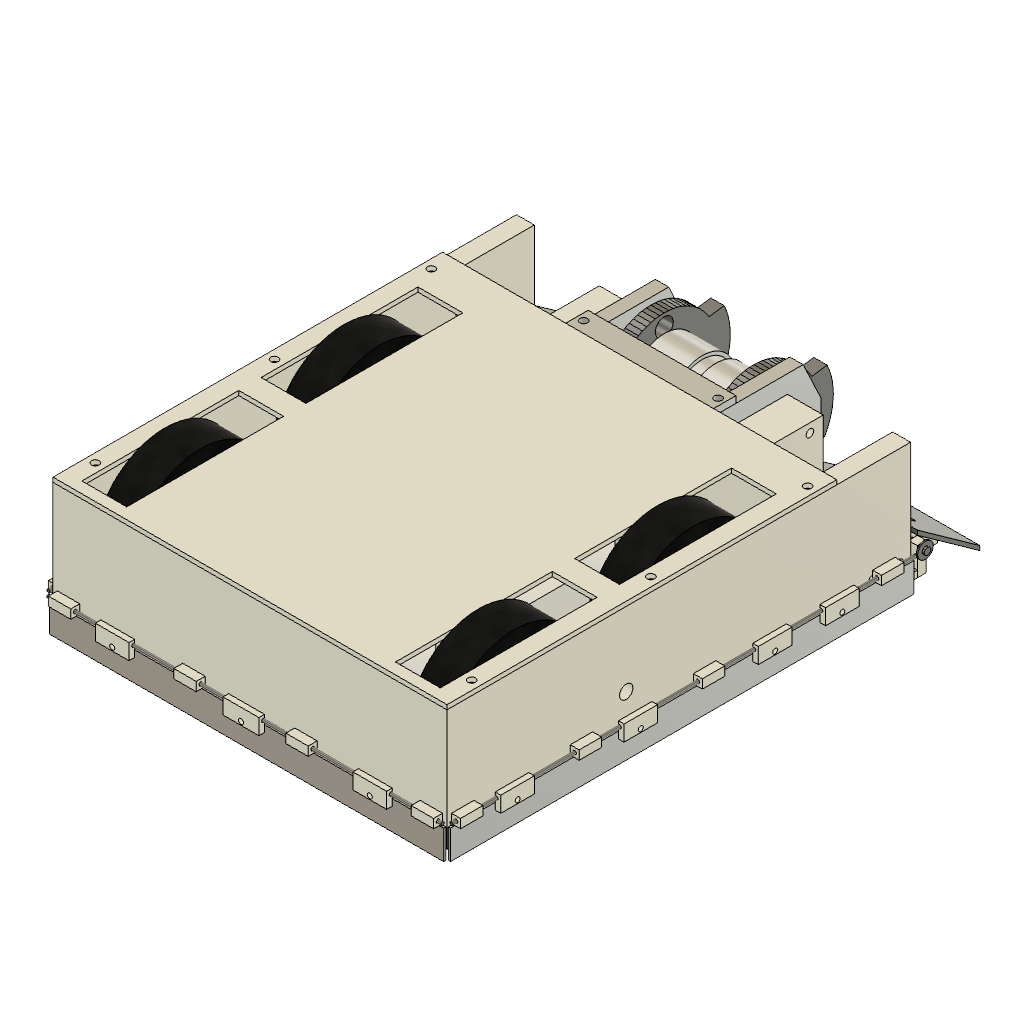
ROBOT_V4_Beater (Autodesk Fusion 360 design; units mm, degrees)
part number: 2026-10-03-23-02-07-533
part number: 2026-10-03-23-02-07-742
part number: 2026-10-03-23-02-07-825
part number: 2026-10-03-23-02-08-845
part number: 2026-10-03-23-02-09-094
part number: 2026-10-03-23-02-09-103
part number: 2026-10-03-23-02-09-172
part number: 2026-10-03-23-02-09-236
part number: 2026-10-03-23-02-09-311
part number: 2026-10-03-23-02-09-393
part number: 2026-10-03-23-02-09-746
part number: 2026-10-03-23-02-10-052
part number: 2026-10-03-23-02-10-324
part number: 2026-10-03-23-02-10-365
part number: 2026-10-03-23-02-10-407
part number: 2026-10-03-23-02-10-450
part number: 2026-10-03-23-02-10-494
part number: 2026-10-03-23-02-10-539
part number: 2026-10-03-23-02-10-582
part number: 2026-10-03-23-02-10-687
part number: 2026-10-03-23-02-10-740
part number: 2026-10-03-23-02-10-976
part number: 2026-10-03-23-02-11-027
part number: 2026-10-03-23-02-11-079
part number: 2026-10-03-23-02-11-094
part number: 2026-10-03-23-02-11-260
part number: 2026-10-03-23-02-11-385
part number: 2026-10-03-23-02-11-847
part number: 2026-10-03-23-02-12-017
part number: 2026-10-03-23-02-12-191
part number: 2026-10-03-23-02-12-302
part number: 2026-10-03-23-02-12-373
part number: 2026-10-03-23-02-12-902
part number: 2026-10-03-23-02-13-104
part number: 2026-10-03-23-02-14-285
part number: 2026-10-03-23-02-14-424
part number: 2026-10-03-23-02-14-508
part number: 2026-10-03-23-02-14-531
part number: 2026-10-03-23-02-14-614
part number: 2026-10-03-23-02-15-140
part number: 2026-10-03-23-02-15-408
part number: 2026-10-03-23-02-15-682
part number: 2026-10-03-23-02-15-969
part number: 2026-10-03-23-02-16-272
part number: 2026-10-03-23-02-16-375
part number: 2026-10-03-23-02-16-912
part number: 2026-10-03-23-02-17-232
part number: 2026-10-03-23-02-17-564
part number: 2026-10-03-23-02-17-904
part number: 2026-10-03-23-02-18-255
part number: 2026-10-03-23-02-18-371
part number: 2026-10-03-23-02-19-002
part number: 2026-10-03-23-02-19-385
part number: 2026-10-03-23-02-19-768
part number: 2026-10-03-23-02-20-163
part number: 2026-10-03-23-02-20-204
part number: 2026-10-03-23-02-20-339
part number: 2026-10-03-23-02-20-844
part number: 2026-10-03-23-02-20-994
part number: 2026-10-03-23-02-21-141
part number: 2026-10-03-23-02-21-679
part number: 2026-10-03-23-02-21-843
part number: 2026-10-03-23-02-22-015
part number: 2026-10-03-23-02-22-630
part number: 2026-10-03-23-02-22-845
part number: 2026-10-03-23-02-23-035
part number: 2026-10-03-23-02-23-656
part number: 2026-10-03-23-02-23-827
part number: 2026-10-03-23-02-23-873
part number: 2026-10-03-23-02-24-050
part number: 2026-10-03-23-02-24-210
part number: 2026-10-03-23-02-24-370
part number: 2026-10-03-23-02-24-531
part number: 2026-10-03-23-02-24-696
part number: 2026-10-03-23-02-24-861
part number: 2026-10-03-23-02-25-025
part number: 2026-10-03-23-02-25-193
part number: 2026-10-03-23-02-25-361
Autodesk Fusion 360 part; units mm, degrees
(part 1 of 3)
sketch "Sketch1" plane through (0, 0, 0) normal (0, 1, 0) x (1, 0, 0) in component "Tub_TPU"
  line L0 (-88, -110) -> (88, -110)
  line L1 (88, -110) -> (88, 64)
  line L2 (88, 64) -> (-88, 64)
  line L3 (-88, 64) -> (-88, -110)
extrude "Extrude1" add sketch "Sketch1" along normal blind 3 from surface at 4 makes body 1 in component "Tub_TPU"
sketch "Floor_WheelWell" plane through (0, 0, 0) normal (1, 0, 0) x (0, 0, -1) in component "Tub_TPU"
  line L0 (-25, 3) -> (-25, 8)
  line L1 (-25, 8) -> (45, 8)
  line L2 (45, 8) -> (45, 3)
  line L3 (45, 3) -> (-25, 3)
extrude "Extrude2" cut sketch "Floor_WheelWell" along normal blind 20 from surface at -80 bodies 1 in component "Tub_TPU"
sketch "Floor_WheelWell (1)" plane through (0, 0, 0) normal (1, 0, 0) x (0, 0, -1) in component "Tub_TPU"
  line L0 (-105, 3) -> (-105, 8)
  line L1 (-105, 8) -> (-35, 8)
  line L2 (-35, 8) -> (-35, 3)
  line L3 (-35, 3) -> (-105, 3)
extrude "Extrude3" cut sketch "Floor_WheelWell (1)" along normal blind 20 from surface at -80 bodies 1 in component "Tub_TPU"
sketch "Floor_WheelWell (2)" plane through (0, 0, 0) normal (1, 0, 0) x (0, 0, -1) in component "Tub_TPU"
  line L0 (-25, 3) -> (-25, 8)
  line L1 (-25, 8) -> (45, 8)
  line L2 (45, 8) -> (45, 3)
  line L3 (45, 3) -> (-25, 3)
extrude "Extrude4" cut sketch "Floor_WheelWell (2)" along normal blind 20 from surface at 60 bodies 1 in component "Tub_TPU"
sketch "Floor_WheelWell (3)" plane through (0, 0, 0) normal (1, 0, 0) x (0, 0, -1) in component "Tub_TPU"
  line L0 (-105, 3) -> (-105, 8)
  line L1 (-105, 8) -> (-35, 8)
  line L2 (-35, 8) -> (-35, 3)
  line L3 (-35, 3) -> (-105, 3)
extrude "Extrude5" cut sketch "Floor_WheelWell (3)" along normal blind 20 from surface at 60 bodies 1 in component "Tub_TPU"
sketch "Side_Wall" plane through (0, 0, 0) normal (1, 0, 0) x (0, 0, -1) in component "Tub_TPU"
  line L0 (-110, 7) -> (-110, 58)
  line L1 (-110, 58) -> (97, 58)
  line L2 (97, 58) -> (97, 7)
  line L3 (97, 7) -> (-110, 7)
extrude "Extrude6" add sketch "Side_Wall" along normal blind 8 from surface at -88 bodies 1 in component "Tub_TPU"
sketch "Side_Wall (1)" plane through (0, 0, 0) normal (1, 0, 0) x (0, 0, -1) in component "Tub_TPU"
  line L0 (-110, 7) -> (-110, 58)
  line L1 (-110, 58) -> (97, 58)
  line L2 (97, 58) -> (97, 7)
  line L3 (97, 7) -> (-110, 7)
extrude "Extrude7" add sketch "Side_Wall (1)" along normal blind 8 from surface at 80 bodies 1 in component "Tub_TPU"
sketch "Rear_Wall" plane through (0, 0, 0) normal (1, 0, 0) x (0, 0, -1) in component "Tub_TPU"
  line L0 (-110, 7) -> (-110, 58)
  line L1 (-110, 58) -> (-104, 58)
  line L2 (-104, 58) -> (-104, 7)
  line L3 (-104, 7) -> (-110, 7)
extrude "Extrude8" add sketch "Rear_Wall" along normal blind 160 from surface at -80 bodies 1 in component "Tub_TPU"
sketch "Front_Bulkhead" plane through (0, 0, 0) normal (1, 0, 0) x (0, 0, -1) in component "Tub_TPU"
  line L0 (62, 7) -> (62, 58)
  line L1 (62, 58) -> (64, 58)
  line L2 (64, 58) -> (64, 7)
  line L3 (64, 7) -> (62, 7)
extrude "Extrude9" add sketch "Front_Bulkhead" along normal blind 160 from surface at -80 bodies 1 in component "Tub_TPU"
sketch "Belt_Slot" plane through (0, 0, 0) normal (1, 0, 0) x (0, 0, -1) in component "Tub_TPU"
  line L0 (61, 12) -> (61, 52)
  line L1 (61, 52) -> (65, 52)
  line L2 (65, 52) -> (65, 12)
  line L3 (65, 12) -> (61, 12)
extrude "Extrude10" cut sketch "Belt_Slot" along normal blind 12 from surface at -6 bodies 1 in component "Tub_TPU"
sketch "Motor_Wall" plane through (0, 0, 0) normal (1, 0, 0) x (0, 0, -1) in component "Tub_TPU"
  line L0 (-3, 7) -> (-3, 58)
  line L1 (-3, 58) -> (23, 58)
  line L2 (23, 58) -> (23, 7)
  line L3 (23, 7) -> (-3, 7)
extrude "Extrude11" add sketch "Motor_Wall" along normal blind 4 from surface at -60 bodies 1 in component "Tub_TPU"
sketch "Motor_Wall (1)" plane through (0, 0, 0) normal (1, 0, 0) x (0, 0, -1) in component "Tub_TPU"
  line L0 (-3, 7) -> (-3, 58)
  line L1 (-3, 58) -> (23, 58)
  line L2 (23, 58) -> (23, 7)
  line L3 (23, 7) -> (-3, 7)
extrude "Extrude12" add sketch "Motor_Wall (1)" along normal blind 4 from surface at 56 bodies 1 in component "Tub_TPU"
sketch "Motor_Shaft_Hole" plane through (0, 0, 0) normal (1, 0, 0) x (0, 0, -1) in component "Tub_TPU"
  circle A0 centre (10, 32) radius 4
extrude "Extrude13" cut sketch "Motor_Shaft_Hole" along normal blind 6 from surface at -61 bodies 1 in component "Tub_TPU"
sketch "Motor_Shaft_Hole (1)" plane through (0, 0, 0) normal (1, 0, 0) x (0, 0, -1) in component "Tub_TPU"
  circle A0 centre (10, 32) radius 4
extrude "Extrude14" cut sketch "Motor_Shaft_Hole (1)" along normal blind 6 from surface at 55 bodies 1 in component "Tub_TPU"
sketch "Motor_Wall (2)" plane through (0, 0, 0) normal (1, 0, 0) x (0, 0, -1) in component "Tub_TPU"
  line L0 (-83, 7) -> (-83, 58)
  line L1 (-83, 58) -> (-57, 58)
  line L2 (-57, 58) -> (-57, 7)
  line L3 (-57, 7) -> (-83, 7)
extrude "Extrude15" add sketch "Motor_Wall (2)" along normal blind 4 from surface at -60 bodies 1 in component "Tub_TPU"
sketch "Motor_Wall (3)" plane through (0, 0, 0) normal (1, 0, 0) x (0, 0, -1) in component "Tub_TPU"
  line L0 (-83, 7) -> (-83, 58)
  line L1 (-83, 58) -> (-57, 58)
  line L2 (-57, 58) -> (-57, 7)
  line L3 (-57, 7) -> (-83, 7)
extrude "Extrude16" add sketch "Motor_Wall (3)" along normal blind 4 from surface at 56 bodies 1 in component "Tub_TPU"
sketch "Motor_Shaft_Hole (2)" plane through (0, 0, 0) normal (1, 0, 0) x (0, 0, -1) in component "Tub_TPU"
  circle A0 centre (-70, 32) radius 4
extrude "Extrude17" cut sketch "Motor_Shaft_Hole (2)" along normal blind 6 from surface at -61 bodies 1 in component "Tub_TPU"
sketch "Motor_Shaft_Hole (3)" plane through (0, 0, 0) normal (1, 0, 0) x (0, 0, -1) in component "Tub_TPU"
  circle A0 centre (-70, 32) radius 4
extrude "Extrude18" cut sketch "Motor_Shaft_Hole (3)" along normal blind 6 from surface at 55 bodies 1 in component "Tub_TPU"
sketch "Front_Floor" plane through (0, 0, 0) normal (1, 0, 0) x (0, 0, -1) in component "Tub_TPU"
  line L0 (64, 4) -> (64, 7)
  line L1 (64, 7) -> (100, 7)
  line L2 (100, 7) -> (100, 4)
  line L3 (100, 4) -> (64, 4)
extrude "Extrude19" add sketch "Front_Floor" along normal blind 54 from surface at -88 bodies 1 in component "Tub_TPU"
sketch "Front_Floor (1)" plane through (0, 0, 0) normal (1, 0, 0) x (0, 0, -1) in component "Tub_TPU"
  line L0 (64, 4) -> (64, 7)
  line L1 (64, 7) -> (100, 7)
  line L2 (100, 7) -> (100, 4)
  line L3 (100, 4) -> (64, 4)
extrude "Extrude20" add sketch "Front_Floor (1)" along normal blind 54 from surface at 34 bodies 1 in component "Tub_TPU"
sketch "Block_Screw_Clearance" plane through (0, 0, 0) normal (1, 0, 0) x (0, 0, -1) in component "Tub_TPU"
  circle A0 centre (80, 13.5) radius 1.7
extrude "Extrude21" cut sketch "Block_Screw_Clearance" along normal blind 10 from surface at -89 bodies 1 in component "Tub_TPU"
sketch "Block_Screw_Clearance (1)" plane through (0, 0, 0) normal (1, 0, 0) x (0, 0, -1) in component "Tub_TPU"
  circle A0 centre (92, 13.5) radius 1.7
extrude "Extrude22" cut sketch "Block_Screw_Clearance (1)" along normal blind 10 from surface at -89 bodies 1 in component "Tub_TPU"
sketch "Block_Screw_Clearance (2)" plane through (0, 0, 0) normal (1, 0, 0) x (0, 0, -1) in component "Tub_TPU"
  circle A0 centre (80, 13.5) radius 1.7
extrude "Extrude23" cut sketch "Block_Screw_Clearance (2)" along normal blind 10 from surface at 79 bodies 1 in component "Tub_TPU"
sketch "Block_Screw_Clearance (3)" plane through (0, 0, 0) normal (1, 0, 0) x (0, 0, -1) in component "Tub_TPU"
  circle A0 centre (92, 13.5) radius 1.7
extrude "Extrude24" cut sketch "Block_Screw_Clearance (3)" along normal blind 10 from surface at 79 bodies 1 in component "Tub_TPU"
sketch "Weapon_Side_Block" plane through (0, 0, 0) normal (1, 0, 0) x (0, 0, -1) in component "Tub_TPU"
  line L0 (64, 7) -> (64, 50)
  line L1 (64, 50) -> (96, 50)
  line L2 (96, 50) -> (96, 7)
  line L3 (96, 7) -> (64, 7)
extrude "Extrude25" add sketch "Weapon_Side_Block" along normal blind 16 from surface at -50 bodies 1 in component "Tub_TPU"
sketch "Upright_Screw_Clearance" plane through (0, 0, 0) normal (1, 0, 0) x (0, 0, -1) in component "Tub_TPU"
  circle A0 centre (70, 14) radius 1.7
extrude "Extrude26" cut sketch "Upright_Screw_Clearance" along normal blind 18 from surface at -51 bodies 1 in component "Tub_TPU"
sketch "Upright_Screw_Clearance (1)" plane through (0, 0, 0) normal (1, 0, 0) x (0, 0, -1) in component "Tub_TPU"
  circle A0 centre (70, 50) radius 1.7
extrude "Extrude27" cut sketch "Upright_Screw_Clearance (1)" along normal blind 18 from surface at -51 bodies 1 in component "Tub_TPU"
sketch "Upright_Screw_Clearance (2)" plane through (0, 0, 0) normal (1, 0, 0) x (0, 0, -1) in component "Tub_TPU"
  circle A0 centre (90, 14) radius 1.7
extrude "Extrude28" cut sketch "Upright_Screw_Clearance (2)" along normal blind 18 from surface at -51 bodies 1 in component "Tub_TPU"
sketch "Upright_Screw_Clearance (3)" plane through (0, 0, 0) normal (1, 0, 0) x (0, 0, -1) in component "Tub_TPU"
  circle A0 centre (90, 46) radius 1.7
extrude "Extrude29" cut sketch "Upright_Screw_Clearance (3)" along normal blind 18 from surface at -51 bodies 1 in component "Tub_TPU"
sketch "Weapon_Side_Block (1)" plane through (0, 0, 0) normal (1, 0, 0) x (0, 0, -1) in component "Tub_TPU"
  line L0 (64, 7) -> (64, 50)
  line L1 (64, 50) -> (96, 50)
  line L2 (96, 50) -> (96, 7)
  line L3 (96, 7) -> (64, 7)
extrude "Extrude30" add sketch "Weapon_Side_Block (1)" along normal blind 16 from surface at 34 bodies 1 in component "Tub_TPU"
sketch "Upright_Screw_Clearance (4)" plane through (0, 0, 0) normal (1, 0, 0) x (0, 0, -1) in component "Tub_TPU"
  circle A0 centre (70, 14) radius 1.7
extrude "Extrude31" cut sketch "Upright_Screw_Clearance (4)" along normal blind 18 from surface at 33 bodies 1 in component "Tub_TPU"
sketch "Upright_Screw_Clearance (5)" plane through (0, 0, 0) normal (1, 0, 0) x (0, 0, -1) in component "Tub_TPU"
  circle A0 centre (70, 50) radius 1.7
extrude "Extrude32" cut sketch "Upright_Screw_Clearance (5)" along normal blind 18 from surface at 33 bodies 1 in component "Tub_TPU"
sketch "Upright_Screw_Clearance (6)" plane through (0, 0, 0) normal (1, 0, 0) x (0, 0, -1) in component "Tub_TPU"
  circle A0 centre (90, 14) radius 1.7
extrude "Extrude33" cut sketch "Upright_Screw_Clearance (6)" along normal blind 18 from surface at 33 bodies 1 in component "Tub_TPU"
sketch "Upright_Screw_Clearance (7)" plane through (0, 0, 0) normal (1, 0, 0) x (0, 0, -1) in component "Tub_TPU"
  circle A0 centre (90, 46) radius 1.7
extrude "Extrude34" cut sketch "Upright_Screw_Clearance (7)" along normal blind 18 from surface at 33 bodies 1 in component "Tub_TPU"
sketch "Lid_Insert" plane through (0, 0, 0) normal (0, 1, 0) x (1, 0, 0) in component "Tub_TPU"
  circle A0 centre (-84, -95) radius 2
extrude "Extrude35" cut sketch "Lid_Insert" along normal blind 8 from surface at 51 bodies 1 in component "Tub_TPU"
sketch "Lid_Insert (1)" plane through (0, 0, 0) normal (0, 1, 0) x (1, 0, 0) in component "Tub_TPU"
  circle A0 centre (-84, -15) radius 2
extrude "Extrude36" cut sketch "Lid_Insert (1)" along normal blind 8 from surface at 51 bodies 1 in component "Tub_TPU"
sketch "Lid_Insert (2)" plane through (0, 0, 0) normal (0, 1, 0) x (1, 0, 0) in component "Tub_TPU"
  circle A0 centre (-84, 55) radius 2
extrude "Extrude37" cut sketch "Lid_Insert (2)" along normal blind 8 from surface at 51 bodies 1 in component "Tub_TPU"
sketch "Lid_Insert (3)" plane through (0, 0, 0) normal (0, 1, 0) x (1, 0, 0) in component "Tub_TPU"
  circle A0 centre (84, -95) radius 2
extrude "Extrude38" cut sketch "Lid_Insert (3)" along normal blind 8 from surface at 51 bodies 1 in component "Tub_TPU"
sketch "Lid_Insert (4)" plane through (0, 0, 0) normal (0, 1, 0) x (1, 0, 0) in component "Tub_TPU"
  circle A0 centre (84, -15) radius 2
extrude "Extrude39" cut sketch "Lid_Insert (4)" along normal blind 8 from surface at 51 bodies 1 in component "Tub_TPU"
sketch "Lid_Insert (5)" plane through (0, 0, 0) normal (0, 1, 0) x (1, 0, 0) in component "Tub_TPU"
  circle A0 centre (84, 55) radius 2
extrude "Extrude40" cut sketch "Lid_Insert (5)" along normal blind 8 from surface at 51 bodies 1 in component "Tub_TPU"
sketch "Switch_Key_Hole" plane through (0, 0, 0) normal (1, 0, 0) x (0, 0, -1) in component "Tub_TPU"
  circle A0 centre (-30, 25) radius 3
extrude "Extrude41" cut sketch "Switch_Key_Hole" along normal blind 10 from surface at 79 bodies 1 in component "Tub_TPU"
sketch "Sketch1 (2)" plane through (0, 0, 0) normal (0, 1, 0) x (1, 0, 0) in component "Lid_TPU_2mm"
  line L0 (-88, -110) -> (88, -110)
  line L1 (88, -110) -> (88, 64)
  line L2 (88, 64) -> (-88, 64)
  line L3 (-88, 64) -> (-88, -110)
extrude "Extrude1'" add sketch "Sketch1 (2)" along normal blind 2 from surface at 58 separate body makes body 2 in component "Lid_TPU_2mm"
sketch "Lid_WheelWell" plane through (0, 0, 0) normal (1, 0, 0) x (0, 0, -1) in component "Lid_TPU_2mm"
  line L0 (-25, 57) -> (-25, 61)
  line L1 (-25, 61) -> (45, 61)
  line L2 (45, 61) -> (45, 57)
  line L3 (45, 57) -> (-25, 57)
extrude "Extrude2'" cut sketch "Lid_WheelWell" along normal blind 20 from surface at -80 bodies 2 in component "Lid_TPU_2mm"
sketch "Lid_WheelWell (1)" plane through (0, 0, 0) normal (1, 0, 0) x (0, 0, -1) in component "Lid_TPU_2mm"
  line L0 (-105, 57) -> (-105, 61)
  line L1 (-105, 61) -> (-35, 61)
  line L2 (-35, 61) -> (-35, 57)
  line L3 (-35, 57) -> (-105, 57)
extrude "Extrude3'" cut sketch "Lid_WheelWell (1)" along normal blind 20 from surface at -80 bodies 2 in component "Lid_TPU_2mm"
sketch "Lid_WheelWell (2)" plane through (0, 0, 0) normal (1, 0, 0) x (0, 0, -1) in component "Lid_TPU_2mm"
  line L0 (-25, 57) -> (-25, 61)
  line L1 (-25, 61) -> (45, 61)
  line L2 (45, 61) -> (45, 57)
  line L3 (45, 57) -> (-25, 57)
extrude "Extrude4'" cut sketch "Lid_WheelWell (2)" along normal blind 20 from surface at 60 bodies 2 in component "Lid_TPU_2mm"
sketch "Lid_WheelWell (3)" plane through (0, 0, 0) normal (1, 0, 0) x (0, 0, -1) in component "Lid_TPU_2mm"
  line L0 (-105, 57) -> (-105, 61)
  line L1 (-105, 61) -> (-35, 61)
  line L2 (-35, 61) -> (-35, 57)
  line L3 (-35, 57) -> (-105, 57)
extrude "Extrude5'" cut sketch "Lid_WheelWell (3)" along normal blind 20 from surface at 60 bodies 2 in component "Lid_TPU_2mm"
sketch "Lid_Screw" plane through (0, 0, 0) normal (0, 1, 0) x (1, 0, 0) in component "Lid_TPU_2mm"
  circle A0 centre (-84, -95) radius 1.7
extrude "Extrude6'" cut sketch "Lid_Screw" along normal blind 4 from surface at 57 bodies 2 in component "Lid_TPU_2mm"
sketch "Lid_Screw (1)" plane through (0, 0, 0) normal (0, 1, 0) x (1, 0, 0) in component "Lid_TPU_2mm"
  circle A0 centre (-84, -15) radius 1.7
extrude "Extrude7'" cut sketch "Lid_Screw (1)" along normal blind 4 from surface at 57 bodies 2 in component "Lid_TPU_2mm"
sketch "Lid_Screw (2)" plane through (0, 0, 0) normal (0, 1, 0) x (1, 0, 0) in component "Lid_TPU_2mm"
  circle A0 centre (-84, 55) radius 1.7
extrude "Extrude8'" cut sketch "Lid_Screw (2)" along normal blind 4 from surface at 57 bodies 2 in component "Lid_TPU_2mm"
sketch "Lid_Screw (3)" plane through (0, 0, 0) normal (0, 1, 0) x (1, 0, 0) in component "Lid_TPU_2mm"
  circle A0 centre (84, -95) radius 1.7
extrude "Extrude9'" cut sketch "Lid_Screw (3)" along normal blind 4 from surface at 57 bodies 2 in component "Lid_TPU_2mm"
sketch "Lid_Screw (4)" plane through (0, 0, 0) normal (0, 1, 0) x (1, 0, 0) in component "Lid_TPU_2mm"
  circle A0 centre (84, -15) radius 1.7
extrude "Extrude10'" cut sketch "Lid_Screw (4)" along normal blind 4 from surface at 57 bodies 2 in component "Lid_TPU_2mm"
sketch "Lid_Screw (5)" plane through (0, 0, 0) normal (0, 1, 0) x (1, 0, 0) in component "Lid_TPU_2mm"
  circle A0 centre (84, 55) radius 1.7
extrude "Extrude11'" cut sketch "Lid_Screw (5)" along normal blind 4 from surface at 57 bodies 2 in component "Lid_TPU_2mm"
sketch "Upright_6061_6mm_L" plane through (0, 0, 0) normal (1, 0, 0) x (0, 0, -1) in component "Upright_6061_6mm_L"
  line L0 (64, 7) -> (64, 57)
  line L1 (64, 57) -> (104, 57)
  line L2 (104, 57) -> (112, 40)
  line L3 (112, 40) -> (112, 16.5)
  line L4 (112, 16.5) -> (100, 25)
  line L5 (100, 25) -> (98, 25)
  line L6 (98, 25) -> (98, 7)
  line L7 (98, 7) -> (64, 7)
  circle A0 centre (95, 32) radius 4.1
  circle A1 centre (70, 14) radius 1.25
  circle A2 centre (70, 50) radius 1.25
  circle A3 centre (90, 14) radius 1.25
  circle A4 centre (90, 46) radius 1.25
extrude "Extrude1''" add sketch "Upright_6061_6mm_L" along normal blind 6 from surface at -33 separate body makes body 3 in component "Upright_6061_6mm_L"
sketch "Upright_6061_6mm_R" plane through (0, 0, 0) normal (1, 0, 0) x (0, 0, -1) in component "Upright_6061_6mm_R"
  line L0 (64, 7) -> (64, 57)
  line L1 (64, 57) -> (104, 57)
  line L2 (104, 57) -> (112, 40)
  line L3 (112, 40) -> (112, 16.5)
  line L4 (112, 16.5) -> (100, 25)
  line L5 (100, 25) -> (98, 25)
  line L6 (98, 25) -> (98, 7)
  line L7 (98, 7) -> (64, 7)
  circle A0 centre (95, 32) radius 4.1
  circle A1 centre (70, 14) radius 1.25
  circle A2 centre (70, 50) radius 1.25
  circle A3 centre (90, 14) radius 1.25
  circle A4 centre (90, 46) radius 1.25
extrude "Extrude1'''" add sketch "Upright_6061_6mm_R" along normal blind 6 from surface at 27 separate body makes body 4 in component "Upright_6061_6mm_R"
sketch "Sketch1 (3)" plane through (0, 0, 0) normal (0, 1, 0) x (1, 0, 0) in component "Weapon_Top_Brace_3mm"
  line L0 (-33, 64) -> (33, 64)
  line L1 (33, 64) -> (33, 74)
  line L2 (33, 74) -> (-33, 74)
  line L3 (-33, 74) -> (-33, 64)
extrude "Extrude1''''" add sketch "Sketch1 (3)" along normal blind 3 from surface at 57 separate body makes body 5 in component "Weapon_Top_Brace_3mm"
sketch "Weapon_Top_Brace_3mm_Hole" plane through (0, 0, 0) normal (0, 1, 0) x (1, 0, 0) in component "Weapon_Top_Brace_3mm"
  circle A0 centre (-30, 69) radius 1.7
extrude "Extrude2''" cut sketch "Weapon_Top_Brace_3mm_Hole" along normal blind 5 from surface at 56 bodies 5 in component "Weapon_Top_Brace_3mm"
sketch "Weapon_Top_Brace_3mm_Hole (1)" plane through (0, 0, 0) normal (0, 1, 0) x (1, 0, 0) in component "Weapon_Top_Brace_3mm"
  circle A0 centre (30, 69) radius 1.7
extrude "Extrude3''" cut sketch "Weapon_Top_Brace_3mm_Hole (1)" along normal blind 5 from surface at 56 bodies 5 in component "Weapon_Top_Brace_3mm"
sketch "Sketch1 (4)" plane through (0, 0, 0) normal (0, 1, 0) x (1, 0, 0) in component "Weapon_Bottom_Brace_3mm"
  line L0 (-33, 64) -> (33, 64)
  line L1 (33, 64) -> (33, 74)
  line L2 (33, 74) -> (-33, 74)
  line L3 (-33, 74) -> (-33, 64)
extrude "Extrude1'''''" add sketch "Sketch1 (4)" along normal blind 3 from surface at 4 separate body makes body 6 in component "Weapon_Bottom_Brace_3mm"
sketch "Weapon_Bottom_Brace_3mm_Hole" plane through (0, 0, 0) normal (0, 1, 0) x (1, 0, 0) in component "Weapon_Bottom_Brace_3mm"
  circle A0 centre (-30, 69) radius 1.7
extrude "Extrude2'''" cut sketch "Weapon_Bottom_Brace_3mm_Hole" along normal blind 5 from surface at 3 bodies 6 in component "Weapon_Bottom_Brace_3mm"
sketch "Weapon_Bottom_Brace_3mm_Hole (1)" plane through (0, 0, 0) normal (0, 1, 0) x (1, 0, 0) in component "Weapon_Bottom_Brace_3mm"
  circle A0 centre (30, 69) radius 1.7
extrude "Extrude3'''" cut sketch "Weapon_Bottom_Brace_3mm_Hole (1)" along normal blind 5 from surface at 3 bodies 6 in component "Weapon_Bottom_Brace_3mm"
sketch "Beater_Disc_L" plane through (0, 0, 0) normal (1, 0, 0) x (0, 0, -1) in component "Beater_Disc_L"
  line L0 (124.5, 32) -> (124.3877, 34.5711)
  line L1 (124.3877, 34.5711) -> (124.0518, 37.1226)
  line L2 (124.0518, 37.1226) -> (123.4948, 39.6352)
  line L3 (123.4948, 39.6352) -> (122.7209, 42.0896)
  line L4 (122.7209, 42.0896) -> (121.7361, 44.4672)
  line L5 (121.7361, 44.4672) -> (114.9186, 43.5)
  line L6 (114.9186, 43.5) -> (113.8405, 45.1923)
  line L7 (113.8405, 45.1923) -> (112.619, 46.7841)
  line L8 (112.619, 46.7841) -> (111.2635, 48.2635)
  line L9 (111.2635, 48.2635) -> (109.7841, 49.619)
  line L10 (109.7841, 49.619) -> (108.1923, 50.8405)
  line L11 (108.1923, 50.8405) -> (106.5, 51.9186)
  line L12 (106.5, 51.9186) -> (104.7202, 52.8451)
  line L13 (104.7202, 52.8451) -> (102.8665, 53.6129)
  line L14 (102.8665, 53.6129) -> (100.9528, 54.2163)
  line L15 (100.9528, 54.2163) -> (98.9939, 54.6506)
  line L16 (98.9939, 54.6506) -> (97.0046, 54.9125)
  line L17 (97.0046, 54.9125) -> (95, 55)
  line L18 (95, 55) -> (92.9954, 54.9125)
  line L19 (92.9954, 54.9125) -> (91.0061, 54.6506)
  line L20 (91.0061, 54.6506) -> (89.0472, 54.2163)
  line L21 (89.0472, 54.2163) -> (87.1335, 53.6129)
  line L22 (87.1335, 53.6129) -> (85.2798, 52.8451)
  line L23 (85.2798, 52.8451) -> (83.5, 51.9186)
  line L24 (83.5, 51.9186) -> (81.8077, 50.8405)
  line L25 (81.8077, 50.8405) -> (80.2159, 49.619)
  line L26 (80.2159, 49.619) -> (78.7365, 48.2635)
  line L27 (78.7365, 48.2635) -> (77.381, 46.7841)
  line L28 (77.381, 46.7841) -> (76.1595, 45.1923)
  line L29 (76.1595, 45.1923) -> (75.0814, 43.5)
  line L30 (75.0814, 43.5) -> (68.2639, 44.4672)
  line L31 (68.2639, 44.4672) -> (67.2791, 42.0896)
  line L32 (67.2791, 42.0896) -> (66.5052, 39.6352)
  line L33 (66.5052, 39.6352) -> (65.9482, 37.1226)
  line L34 (65.9482, 37.1226) -> (65.6123, 34.5711)
  line L35 (65.6123, 34.5711) -> (65.5, 32)
  line L36 (65.5, 32) -> (65.6123, 29.4289)
  line L37 (65.6123, 29.4289) -> (65.9482, 26.8774)
  line L38 (65.9482, 26.8774) -> (66.5052, 24.3648)
  line L39 (66.5052, 24.3648) -> (67.2791, 21.9104)
  line L40 (67.2791, 21.9104) -> (68.2639, 19.5328)
  line L41 (68.2639, 19.5328) -> (75.0814, 20.5)
  line L42 (75.0814, 20.5) -> (76.1595, 18.8077)
  line L43 (76.1595, 18.8077) -> (77.381, 17.2159)
  line L44 (77.381, 17.2159) -> (78.7365, 15.7365)
  line L45 (78.7365, 15.7365) -> (80.2159, 14.381)
  line L46 (80.2159, 14.381) -> (81.8077, 13.1595)
  line L47 (81.8077, 13.1595) -> (83.5, 12.0814)
  line L48 (83.5, 12.0814) -> (85.2798, 11.1549)
  line L49 (85.2798, 11.1549) -> (87.1335, 10.3871)
  line L50 (87.1335, 10.3871) -> (89.0472, 9.7837)
  line L51 (89.0472, 9.7837) -> (91.0061, 9.3494)
  line L52 (91.0061, 9.3494) -> (92.9954, 9.0875)
  line L53 (92.9954, 9.0875) -> (95, 9)
  line L54 (95, 9) -> (97.0046, 9.0875)
  line L55 (97.0046, 9.0875) -> (98.9939, 9.3494)
  line L56 (98.9939, 9.3494) -> (100.9528, 9.7837)
  line L57 (100.9528, 9.7837) -> (102.8665, 10.3871)
  line L58 (102.8665, 10.3871) -> (104.7202, 11.1549)
  line L59 (104.7202, 11.1549) -> (106.5, 12.0814)
  line L60 (106.5, 12.0814) -> (108.1923, 13.1595)
  line L61 (108.1923, 13.1595) -> (109.7841, 14.381)
  line L62 (109.7841, 14.381) -> (111.2635, 15.7365)
  line L63 (111.2635, 15.7365) -> (112.619, 17.2159)
  line L64 (112.619, 17.2159) -> (113.8405, 18.8077)
  line L65 (113.8405, 18.8077) -> (120.5477, 17.25)
  line L66 (120.5477, 17.25) -> (121.7361, 19.5328)
  line L67 (121.7361, 19.5328) -> (122.7209, 21.9104)
  line L68 (122.7209, 21.9104) -> (123.4948, 24.3648)
  line L69 (123.4948, 24.3648) -> (124.0518, 26.8774)
  line L70 (124.0518, 26.8774) -> (124.3877, 29.4289)
  line L71 (124.3877, 29.4289) -> (124.5, 32)
  circle A0 centre (95, 32) radius 7
  circle A1 centre (104.1924, 41.1924) radius 1.7
  circle A2 centre (85.8076, 41.1924) radius 1.7
  circle A3 centre (85.8076, 22.8076) radius 1.7
  circle A4 centre (104.1924, 22.8076) radius 1.7
  circle A5 centre (95, 49.5) radius 4
  circle A6 centre (95, 14.5) radius 4
extrude "Extrude1''''''" add sketch "Beater_Disc_L" along normal blind 6 from surface at -26 separate body makes body 7 in component "Beater_Disc_L"
sketch "Beater_Disc_R" plane through (0, 0, 0) normal (1, 0, 0) x (0, 0, -1) in component "Beater_Disc_R"
  line L0 (124.5, 32) -> (124.3877, 34.5711)
  line L1 (124.3877, 34.5711) -> (124.0518, 37.1226)
  line L2 (124.0518, 37.1226) -> (123.4948, 39.6352)
  line L3 (123.4948, 39.6352) -> (122.7209, 42.0896)
  line L4 (122.7209, 42.0896) -> (121.7361, 44.4672)
  line L5 (121.7361, 44.4672) -> (114.9186, 43.5)
  line L6 (114.9186, 43.5) -> (113.8405, 45.1923)
  line L7 (113.8405, 45.1923) -> (112.619, 46.7841)
  line L8 (112.619, 46.7841) -> (111.2635, 48.2635)
  line L9 (111.2635, 48.2635) -> (109.7841, 49.619)
  line L10 (109.7841, 49.619) -> (108.1923, 50.8405)
  line L11 (108.1923, 50.8405) -> (106.5, 51.9186)
  line L12 (106.5, 51.9186) -> (104.7202, 52.8451)
  line L13 (104.7202, 52.8451) -> (102.8665, 53.6129)
  line L14 (102.8665, 53.6129) -> (100.9528, 54.2163)
  line L15 (100.9528, 54.2163) -> (98.9939, 54.6506)
  line L16 (98.9939, 54.6506) -> (97.0046, 54.9125)
  line L17 (97.0046, 54.9125) -> (95, 55)
  line L18 (95, 55) -> (92.9954, 54.9125)
  line L19 (92.9954, 54.9125) -> (91.0061, 54.6506)
  line L20 (91.0061, 54.6506) -> (89.0472, 54.2163)
  line L21 (89.0472, 54.2163) -> (87.1335, 53.6129)
  line L22 (87.1335, 53.6129) -> (85.2798, 52.8451)
  line L23 (85.2798, 52.8451) -> (83.5, 51.9186)
  line L24 (83.5, 51.9186) -> (81.8077, 50.8405)
  line L25 (81.8077, 50.8405) -> (80.2159, 49.619)
  line L26 (80.2159, 49.619) -> (78.7365, 48.2635)
  line L27 (78.7365, 48.2635) -> (77.381, 46.7841)
  line L28 (77.381, 46.7841) -> (76.1595, 45.1923)
  line L29 (76.1595, 45.1923) -> (75.0814, 43.5)
  line L30 (75.0814, 43.5) -> (68.2639, 44.4672)
  line L31 (68.2639, 44.4672) -> (67.2791, 42.0896)
  line L32 (67.2791, 42.0896) -> (66.5052, 39.6352)
  line L33 (66.5052, 39.6352) -> (65.9482, 37.1226)
  line L34 (65.9482, 37.1226) -> (65.6123, 34.5711)
  line L35 (65.6123, 34.5711) -> (65.5, 32)
  line L36 (65.5, 32) -> (65.6123, 29.4289)
  line L37 (65.6123, 29.4289) -> (65.9482, 26.8774)
  line L38 (65.9482, 26.8774) -> (66.5052, 24.3648)
  line L39 (66.5052, 24.3648) -> (67.2791, 21.9104)
  line L40 (67.2791, 21.9104) -> (68.2639, 19.5328)
  line L41 (68.2639, 19.5328) -> (75.0814, 20.5)
  line L42 (75.0814, 20.5) -> (76.1595, 18.8077)
  line L43 (76.1595, 18.8077) -> (77.381, 17.2159)
  line L44 (77.381, 17.2159) -> (78.7365, 15.7365)
  line L45 (78.7365, 15.7365) -> (80.2159, 14.381)
  line L46 (80.2159, 14.381) -> (81.8077, 13.1595)
  line L47 (81.8077, 13.1595) -> (83.5, 12.0814)
  line L48 (83.5, 12.0814) -> (85.2798, 11.1549)
  line L49 (85.2798, 11.1549) -> (87.1335, 10.3871)
  line L50 (87.1335, 10.3871) -> (89.0472, 9.7837)
  line L51 (89.0472, 9.7837) -> (91.0061, 9.3494)
  line L52 (91.0061, 9.3494) -> (92.9954, 9.0875)
  line L53 (92.9954, 9.0875) -> (95, 9)
  line L54 (95, 9) -> (97.0046, 9.0875)
  line L55 (97.0046, 9.0875) -> (98.9939, 9.3494)
  line L56 (98.9939, 9.3494) -> (100.9528, 9.7837)
  line L57 (100.9528, 9.7837) -> (102.8665, 10.3871)
  line L58 (102.8665, 10.3871) -> (104.7202, 11.1549)
  line L59 (104.7202, 11.1549) -> (106.5, 12.0814)
  line L60 (106.5, 12.0814) -> (108.1923, 13.1595)
  line L61 (108.1923, 13.1595) -> (109.7841, 14.381)
  line L62 (109.7841, 14.381) -> (111.2635, 15.7365)
  line L63 (111.2635, 15.7365) -> (112.619, 17.2159)
  line L64 (112.619, 17.2159) -> (113.8405, 18.8077)
  line L65 (113.8405, 18.8077) -> (120.5477, 17.25)
  line L66 (120.5477, 17.25) -> (121.7361, 19.5328)
  line L67 (121.7361, 19.5328) -> (122.7209, 21.9104)
  line L68 (122.7209, 21.9104) -> (123.4948, 24.3648)
  line L69 (123.4948, 24.3648) -> (124.0518, 26.8774)
  line L70 (124.0518, 26.8774) -> (124.3877, 29.4289)
  line L71 (124.3877, 29.4289) -> (124.5, 32)
  circle A0 centre (95, 32) radius 7
  circle A1 centre (104.1924, 41.1924) radius 1.7
  circle A2 centre (85.8076, 41.1924) radius 1.7
  circle A3 centre (85.8076, 22.8076) radius 1.7
  circle A4 centre (104.1924, 22.8076) radius 1.7
  circle A5 centre (95, 49.5) radius 4
  circle A6 centre (95, 14.5) radius 4
extrude "Extrude1'''''''" add sketch "Beater_Disc_R" along normal blind 6 from surface at 20 separate body makes body 8 in component "Beater_Disc_R"
sketch "Beater_Hub_6061_D30" plane through (0, 0, 0) normal (1, 0, 0) x (0, 0, -1) in component "Beater_Hub_6061_D30"
  circle A0 centre (95, 32) radius 15
  circle A1 centre (95, 32) radius 11
extrude "Extrude1''''''''" add sketch "Beater_Hub_6061_D30" along normal blind 40 from surface at -20 separate body makes body 9 in component "Beater_Hub_6061_D30"
sketch "Belt_Groove" plane through (0, 0, 0) normal (1, 0, 0) x (0, 0, -1) in component "Beater_Hub_6061_D30"
  circle A0 centre (95, 32) radius 15.5
  circle A1 centre (95, 32) radius 13.5
extrude "Extrude2''''" cut sketch "Belt_Groove" along normal blind 6 from surface at -3 bodies 9 in component "Beater_Hub_6061_D30"
sketch "M3_Tap" plane through (0, 0, 0) normal (1, 0, 0) x (0, 0, -1) in component "Beater_Hub_6061_D30"
  circle A0 centre (104.1924, 41.1924) radius 1.25
extrude "Extrude3''''" cut sketch "M3_Tap" along normal blind 8 from surface at -20 bodies 9 in component "Beater_Hub_6061_D30"
sketch "M3_Tap (1)" plane through (0, 0, 0) normal (1, 0, 0) x (0, 0, -1) in component "Beater_Hub_6061_D30"
  circle A0 centre (104.1924, 41.1924) radius 1.25
extrude "Extrude4''" cut sketch "M3_Tap (1)" along normal blind 8 from surface at 12 bodies 9 in component "Beater_Hub_6061_D30"
sketch "M3_Tap (2)" plane through (0, 0, 0) normal (1, 0, 0) x (0, 0, -1) in component "Beater_Hub_6061_D30"
  circle A0 centre (85.8076, 41.1924) radius 1.25
extrude "Extrude5''" cut sketch "M3_Tap (2)" along normal blind 8 from surface at -20 bodies 9 in component "Beater_Hub_6061_D30"
sketch "M3_Tap (3)" plane through (0, 0, 0) normal (1, 0, 0) x (0, 0, -1) in component "Beater_Hub_6061_D30"
  circle A0 centre (85.8076, 41.1924) radius 1.25
extrude "Extrude6''" cut sketch "M3_Tap (3)" along normal blind 8 from surface at 12 bodies 9 in component "Beater_Hub_6061_D30"
sketch "M3_Tap (4)" plane through (0, 0, 0) normal (1, 0, 0) x (0, 0, -1) in component "Beater_Hub_6061_D30"
  circle A0 centre (85.8076, 22.8076) radius 1.25
extrude "Extrude7''" cut sketch "M3_Tap (4)" along normal blind 8 from surface at -20 bodies 9 in component "Beater_Hub_6061_D30"
sketch "M3_Tap (5)" plane through (0, 0, 0) normal (1, 0, 0) x (0, 0, -1) in component "Beater_Hub_6061_D30"
  circle A0 centre (85.8076, 22.8076) radius 1.25
extrude "Extrude8''" cut sketch "M3_Tap (5)" along normal blind 8 from surface at 12 bodies 9 in component "Beater_Hub_6061_D30"
sketch "M3_Tap (6)" plane through (0, 0, 0) normal (1, 0, 0) x (0, 0, -1) in component "Beater_Hub_6061_D30"
  circle A0 centre (104.1924, 22.8076) radius 1.25
extrude "Extrude9''" cut sketch "M3_Tap (6)" along normal blind 8 from surface at -20 bodies 9 in component "Beater_Hub_6061_D30"
sketch "M3_Tap (7)" plane through (0, 0, 0) normal (1, 0, 0) x (0, 0, -1) in component "Beater_Hub_6061_D30"
  circle A0 centre (104.1924, 22.8076) radius 1.25
extrude "Extrude10''" cut sketch "M3_Tap (7)" along normal blind 8 from surface at 12 bodies 9 in component "Beater_Hub_6061_D30"
sketch "Bearing_608_L" plane through (0, 0, 0) normal (1, 0, 0) x (0, 0, -1) in component "Bearing_608_L"
  circle A0 centre (95, 32) radius 11
  circle A1 centre (95, 32) radius 4
extrude "Extrude1'''''''''" add sketch "Bearing_608_L" along normal blind 7 from surface at -20 separate body makes body 10 in component "Bearing_608_L"
sketch "Bearing_608_R" plane through (0, 0, 0) normal (1, 0, 0) x (0, 0, -1) in component "Bearing_608_R"
  circle A0 centre (95, 32) radius 11
  circle A1 centre (95, 32) radius 4
extrude "Extrude1''''''''''" add sketch "Bearing_608_R" along normal blind 7 from surface at 13 separate body makes body 11 in component "Bearing_608_R"
sketch "Spacer_Outer_L_ID8.2_OD11" plane through (0, 0, 0) normal (1, 0, 0) x (0, 0, -1) in component "Spacer_Outer_L_ID8.2_OD11"
  circle A0 centre (95, 32) radius 5.5
  circle A1 centre (95, 32) radius 4.1
extrude "Extrude1'''''''''''" add sketch "Spacer_Outer_L_ID8.2_OD11" along normal blind 7 from surface at -27 separate body makes body 12 in component "Spacer_Outer_L_ID8.2_OD11"
sketch "Spacer_Inner_ID8.2_OD11" plane through (0, 0, 0) normal (1, 0, 0) x (0, 0, -1) in component "Spacer_Inner_ID8.2_OD11"
  circle A0 centre (95, 32) radius 5.5
  circle A1 centre (95, 32) radius 4.1
extrude "Extrude1''''''''''''" add sketch "Spacer_Inner_ID8.2_OD11" along normal blind 26 from surface at -13 separate body makes body 13 in component "Spacer_Inner_ID8.2_OD11"
sketch "Spacer_Outer_R_ID8.2_OD11" plane through (0, 0, 0) normal (1, 0, 0) x (0, 0, -1) in component "Spacer_Outer_R_ID8.2_OD11"
  circle A0 centre (95, 32) radius 5.5
  circle A1 centre (95, 32) radius 4.1
extrude "Extrude1'''''''''''''" add sketch "Spacer_Outer_R_ID8.2_OD11" along normal blind 7 from surface at 20 separate body makes body 14 in component "Spacer_Outer_R_ID8.2_OD11"
sketch "Dead_Shaft_M8_12.9" plane through (0, 0, 0) normal (1, 0, 0) x (0, 0, -1) in component "Dead_Shaft_M8_12.9"
  circle A0 centre (95, 32) radius 4
extrude "Extrude1''''''''''''''" add sketch "Dead_Shaft_M8_12.9" along normal blind 66 from surface at -33 separate body makes body 15 in component "Dead_Shaft_M8_12.9"
sketch "D3536_1250kV_Can_ENVELOPE" plane through (0, 0, 0) normal (1, 0, 0) x (0, 0, -1) in component "D3536_1250kV_Can_ENVELOPE"
  circle A0 centre (44, 32) radius 17.5
extrude "Extrude1'''''''''''''''" add sketch "D3536_1250kV_Can_ENVELOPE" along normal blind 36 from surface at -41 separate body makes body 16 in component "D3536_1250kV_Can_ENVELOPE"
sketch "Motor_Pulley_D26_Groove" plane through (0, 0, 0) normal (1, 0, 0) x (0, 0, -1) in component "Motor_Pulley_D26_Groove"
  circle A0 centre (44, 32) radius 13
  circle A1 centre (44, 32) radius 2.5
extrude "Extrude1''''''''''''''''" add sketch "Motor_Pulley_D26_Groove" along normal blind 8 from surface at -4 separate body makes body 17 in component "Motor_Pulley_D26_Groove"
sketch "Sketch1 (5)" plane through (0, 0, 0) normal (0, 1, 0) x (1, 0, 0) in component "Weapon_Motor_Mount_3mm"
  line L0 (-45, 26) -> (-42, 26)
  line L1 (-42, 26) -> (-42, 62)
  line L2 (-42, 62) -> (-45, 62)
  line L3 (-45, 62) -> (-45, 26)
extrude "Extrude1'''''''''''''''''" add sketch "Sketch1 (5)" along normal blind 44 from surface at 10 separate body makes body 18 in component "Weapon_Motor_Mount_3mm"
sketch "Motor_Centre" plane through (0, 0, 0) normal (1, 0, 0) x (0, 0, -1) in component "Weapon_Motor_Mount_3mm"
  circle A0 centre (44, 32) radius 5
extrude "Extrude2'''''" cut sketch "Motor_Centre" along normal blind 5 from surface at -46 bodies 18 in component "Weapon_Motor_Mount_3mm"
sketch "Motor_M3" plane through (0, 0, 0) normal (1, 0, 0) x (0, 0, -1) in component "Weapon_Motor_Mount_3mm"
  circle A0 centre (36, 32) radius 1.7
extrude "Extrude3'''''" cut sketch "Motor_M3" along normal blind 5 from surface at -46 bodies 18 in component "Weapon_Motor_Mount_3mm"
sketch "Motor_M3 (1)" plane through (0, 0, 0) normal (1, 0, 0) x (0, 0, -1) in component "Weapon_Motor_Mount_3mm"
  circle A0 centre (52, 32) radius 1.7
extrude "Extrude4'''" cut sketch "Motor_M3 (1)" along normal blind 5 from surface at -46 bodies 18 in component "Weapon_Motor_Mount_3mm"
sketch "Motor_M3 (2)" plane through (0, 0, 0) normal (1, 0, 0) x (0, 0, -1) in component "Weapon_Motor_Mount_3mm"
  circle A0 centre (44, 22.5) radius 1.7
extrude "Extrude5'''" cut sketch "Motor_M3 (2)" along normal blind 5 from surface at -46 bodies 18 in component "Weapon_Motor_Mount_3mm"
sketch "Motor_M3 (3)" plane through (0, 0, 0) normal (1, 0, 0) x (0, 0, -1) in component "Weapon_Motor_Mount_3mm"
  circle A0 centre (44, 41.5) radius 1.7
extrude "Extrude6'''" cut sketch "Motor_M3 (3)" along normal blind 5 from surface at -46 bodies 18 in component "Weapon_Motor_Mount_3mm"
sketch "Sketch1 (6)" plane through (0, 0, 0) normal (0, 1, 0) x (1, 0, 0) in component "Belt_Upper_ENVELOPE"
  line L0 (-3, 52) -> (3, 52)
  line L1 (3, 52) -> (3, 86)
  line L2 (3, 86) -> (-3, 86)
  line L3 (-3, 86) -> (-3, 52)
extrude "Extrude1''''''''''''''''''" add sketch "Sketch1 (6)" along normal blind 1.5 from surface at 45.5 separate body makes body 19 in component "Belt_Upper_ENVELOPE"
sketch "Sketch1 (7)" plane through (0, 0, 0) normal (0, 1, 0) x (1, 0, 0) in component "Belt_Lower_ENVELOPE"
  line L0 (-3, 52) -> (3, 52)
  line L1 (3, 52) -> (3, 86)
  line L2 (3, 86) -> (-3, 86)
  line L3 (-3, 86) -> (-3, 52)
extrude "Extrude1'''''''''''''''''''" add sketch "Sketch1 (7)" along normal blind 1.5 from surface at 17 separate body makes body 20 in component "Belt_Lower_ENVELOPE"
sketch "Wedgelet_L" plane through (0, 0, 0) normal (1, 0, 0) x (0, 0, -1) in component "Wedgelet_L"
  line L0 (128, 0.5) -> (128, 2.5)
  line L1 (128, 2.5) -> (100, 22.5)
  line L2 (100, 22.5) -> (100, 20.5)
  line L3 (100, 20.5) -> (128, 0.5)
extrude "Extrude1''''''''''''''''''''" add sketch "Wedgelet_L" along normal blind 61 from surface at -88 separate body makes body 21 in component "Wedgelet_L"
sketch "Wedgelet_M3" plane through (0, 62.1959, -44.4257) normal (0, 0.813733, -0.581238) x (0, 0.581238, 0.813733) in component "Wedgelet_L"
  line L0 (-102.7048, -88) -> (-68.2955, -88)
  line L1 (-68.2955, -88) -> (-68.2955, -27)
  line L2 (-68.2955, -27) -> (-102.7048, -27)
  line L3 (-102.7048, -27) -> (-102.7048, -88)
  circle A0 centre (-80.5845, -49) radius 1.7
  circle A1 centre (-80.5845, -75) radius 1.7
extrude "Extrude2''''''" cut sketch "Wedgelet_M3" along normal mid plane 6 contours A0 | A1 bodies 21 in component "Wedgelet_L"
sketch "Wedgelet_R" plane through (0, 0, 0) normal (1, 0, 0) x (0, 0, -1) in component "Wedgelet_R"
  line L0 (128, 0.5) -> (128, 2.5)
  line L1 (128, 2.5) -> (100, 22.5)
  line L2 (100, 22.5) -> (100, 20.5)
  line L3 (100, 20.5) -> (128, 0.5)
extrude "Extrude1'''''''''''''''''''''" add sketch "Wedgelet_R" along normal blind 61 from surface at 27 separate body makes body 22 in component "Wedgelet_R"
sketch "Wedgelet_M3 (2)" plane through (0, 62.1959, -44.4257) normal (0, 0.813733, -0.581238) x (0, 0.581238, 0.813733) in component "Wedgelet_R"
  line L0 (-102.7048, 27) -> (-68.2955, 27)
  line L1 (-68.2955, 27) -> (-68.2955, 88)
  line L2 (-68.2955, 88) -> (-102.7048, 88)
  line L3 (-102.7048, 88) -> (-102.7048, 27)
  circle A0 centre (-80.5845, 49) radius 1.7
  circle A1 centre (-80.5845, 75) radius 1.7
extrude "Extrude2'''''''" cut sketch "Wedgelet_M3 (2)" along normal mid plane 6 contours A0 | A1 bodies 22 in component "Wedgelet_R"
sketch "Wedgelet_Block_PETG_L" plane through (0, 0, 0) normal (1, 0, 0) x (0, 0, -1) in component "Wedgelet_Block_PETG_L"
  line L0 (100, 4) -> (100, 11)
  line L1 (100, 11) -> (104, 11)
  line L2 (104, 11) -> (104, 4)
  line L3 (104, 4) -> (100, 4)
extrude "Extrude1''''''''''''''''''''''" add sketch "Wedgelet_Block_PETG_L" along normal blind 54 from surface at -88 separate body makes body 23 in component "Wedgelet_Block_PETG_L"
sketch "Knuckle" plane through (0, 0, 0) normal (1, 0, 0) x (0, 0, -1) in component "Wedgelet_Block_PETG_L"
  line L0 (100, 11) -> (100, 16.5)
  line L1 (100, 16.5) -> (104, 16.5)
  line L2 (104, 16.5) -> (104, 11)
  line L3 (104, 11) -> (100, 11)
extrude "Extrude2''''''''" add sketch "Knuckle" along normal blind 4 from surface at -38 bodies 23 in component "Wedgelet_Block_PETG_L"
sketch "Knuckle (1)" plane through (0, 0, 0) normal (1, 0, 0) x (0, 0, -1) in component "Wedgelet_Block_PETG_L"
  line L0 (100, 11) -> (100, 16.5)
  line L1 (100, 16.5) -> (104, 16.5)
  line L2 (104, 16.5) -> (104, 11)
  line L3 (104, 11) -> (100, 11)
extrude "Extrude3''''''" add sketch "Knuckle (1)" along normal blind 6 from surface at -66 bodies 23 in component "Wedgelet_Block_PETG_L"
sketch "Knuckle (2)" plane through (0, 0, 0) normal (1, 0, 0) x (0, 0, -1) in component "Wedgelet_Block_PETG_L"
  line L0 (100, 11) -> (100, 16.5)
  line L1 (100, 16.5) -> (104, 16.5)
  line L2 (104, 16.5) -> (104, 11)
  line L3 (104, 11) -> (100, 11)
extrude "Extrude4''''" add sketch "Knuckle (2)" along normal blind 4 from surface at -88 bodies 23 in component "Wedgelet_Block_PETG_L"
sketch "Bridge" plane through (0, 0, 0) normal (1, 0, 0) x (0, 0, -1) in component "Wedgelet_Block_PETG_L"
  line L0 (97, 7) -> (97, 10)
  line L1 (97, 10) -> (101, 10)
  line L2 (101, 10) -> (101, 7)
  line L3 (101, 7) -> (97, 7)
extrude "Extrude5''''" add sketch "Bridge" along normal blind 10 from surface at -80 bodies 23 in component "Wedgelet_Block_PETG_L"
sketch "Rail" plane through (0, 0, 0) normal (1, 0, 0) x (0, 0, -1) in component "Wedgelet_Block_PETG_L"
  line L0 (64, 7) -> (64, 18)
  line L1 (64, 18) -> (98, 18)
  line L2 (98, 18) -> (98, 7)
  line L3 (98, 7) -> (64, 7)
extrude "Extrude6''''" add sketch "Rail" along normal blind 10 from surface at -80 bodies 23 in component "Wedgelet_Block_PETG_L"
sketch "Pin_Bore" plane through (0, 0, 0) normal (1, 0, 0) x (0, 0, -1) in component "Wedgelet_Block_PETG_L"
  circle A0 centre (102, 14.5) radius 1.6
extrude "Extrude7'''" cut sketch "Pin_Bore" along normal blind 56 from surface at -89 bodies 23 in component "Wedgelet_Block_PETG_L"
sketch "Wall_Insert" plane through (0, 0, 0) normal (1, 0, 0) x (0, 0, -1) in component "Wedgelet_Block_PETG_L"
  circle A0 centre (80, 13.5) radius 2
extrude "Extrude8'''" cut sketch "Wall_Insert" along normal blind 8 from surface at -80 bodies 23 in component "Wedgelet_Block_PETG_L"
sketch "Wall_Insert (1)" plane through (0, 0, 0) normal (1, 0, 0) x (0, 0, -1) in component "Wedgelet_Block_PETG_L"
  circle A0 centre (92, 13.5) radius 2
extrude "Extrude9'''" cut sketch "Wall_Insert (1)" along normal blind 8 from surface at -80 bodies 23 in component "Wedgelet_Block_PETG_L"
sketch "Wedgelet_Carrier_PETG_L1" plane through (0, 0, 0) normal (1, 0, 0) x (0, 0, -1) in component "Wedgelet_Carrier_PETG_L1"
  line L0 (100, 11.5) -> (100, 20.5)
  line L1 (100, 20.5) -> (114, 10.5)
  line L2 (114, 10.5) -> (114, 8)
  line L3 (114, 8) -> (105, 8)
  line L4 (105, 8) -> (104.5, 11.5)
  line L5 (104.5, 11.5) -> (100, 11.5)
extrude "Extrude1'''''''''''''''''''''''" add sketch "Wedgelet_Carrier_PETG_L1" along normal blind 20 from surface at -59 separate body makes body 24 in component "Wedgelet_Carrier_PETG_L1"
sketch "Pin_Bore (2)" plane through (0, 0, 0) normal (1, 0, 0) x (0, 0, -1) in component "Wedgelet_Carrier_PETG_L1"
  circle A0 centre (102, 14.5) radius 1.6
extrude "Extrude2'''''''''" cut sketch "Pin_Bore (2)" along normal blind 22 from surface at -60 bodies 24 in component "Wedgelet_Carrier_PETG_L1"
sketch "Wedgelet_Insert" plane through (0, 60.8716, -43.4797) normal (0, 0.813733, -0.581238) x (0, 0.581238, 0.813733) in component "Wedgelet_Carrier_PETG_L1"
  line L0 (-86.6626, -59) -> (-69.458, -59)
  line L1 (-69.458, -59) -> (-69.458, -39)
  line L2 (-69.458, -39) -> (-86.6626, -39)
  line L3 (-86.6626, -39) -> (-86.6626, -59)
  circle A0 through (-78.5829, -49, -0.0046) (-81.5829, -47.2679, -0.0046) (-81.5829, -50.7321, -0.0046)
extrude "Extrude3'''''''" cut sketch "Wedgelet_Insert" along normal mid plane 12 contours A0 in plane through (0, 60.8679, -43.4771) normal (0, 0.813733, -0.581238) bodies 24 in component "Wedgelet_Carrier_PETG_L1"
sketch "Wedgelet_Carrier_PETG_L2" plane through (0, 0, 0) normal (1, 0, 0) x (0, 0, -1) in component "Wedgelet_Carrier_PETG_L2"
  line L0 (100, 11.5) -> (100, 20.5)
  line L1 (100, 20.5) -> (114, 10.5)
  line L2 (114, 10.5) -> (114, 8)
  line L3 (114, 8) -> (105, 8)
  line L4 (105, 8) -> (104.5, 11.5)
  line L5 (104.5, 11.5) -> (100, 11.5)
extrude "Extrude1''''''''''''''''''''''''" add sketch "Wedgelet_Carrier_PETG_L2" along normal blind 16 from surface at -83 separate body makes body 25 in component "Wedgelet_Carrier_PETG_L2"
sketch "Pin_Bore (3)" plane through (0, 0, 0) normal (1, 0, 0) x (0, 0, -1) in component "Wedgelet_Carrier_PETG_L2"
  circle A0 centre (102, 14.5) radius 1.6
extrude "Extrude2''''''''''" cut sketch "Pin_Bore (3)" along normal blind 18 from surface at -84 bodies 25 in component "Wedgelet_Carrier_PETG_L2"
sketch "Wedgelet_Insert (2)" plane through (0, 60.8716, -43.4797) normal (0, 0.813733, -0.581238) x (0, 0.581238, 0.813733) in component "Wedgelet_Carrier_PETG_L2"
  line L0 (-86.6626, -83) -> (-69.458, -83)
  line L1 (-69.458, -83) -> (-69.458, -67)
  line L2 (-69.458, -67) -> (-86.6626, -67)
  line L3 (-86.6626, -67) -> (-86.6626, -83)
  circle A0 through (-78.5829, -75, -0.0046) (-81.5829, -73.2679, -0.0046) (-81.5829, -76.7321, -0.0046)
extrude "Extrude3''''''''" cut sketch "Wedgelet_Insert (2)" along normal mid plane 12 contours A0 in plane through (0, 60.8679, -43.4771) normal (0, 0.813733, -0.581238) bodies 25 in component "Wedgelet_Carrier_PETG_L2"
sketch "Hinge_Pin_D3_L" plane through (0, 0, 0) normal (1, 0, 0) x (0, 0, -1) in component "Hinge_Pin_D3_L"
  circle A0 centre (102, 14.5) radius 1.5
extrude "Extrude1'''''''''''''''''''''''''" add sketch "Hinge_Pin_D3_L" along normal blind 57 from surface at -90.5 separate body makes body 26 in component "Hinge_Pin_D3_L"
sketch "Eclip_Groove" plane through (0, 0, 0) normal (1, 0, 0) x (0, 0, -1) in component "Hinge_Pin_D3_L"
  circle A0 centre (102, 14.5) radius 1.5
  circle A1 centre (102, 14.5) radius 1.15
extrude "Extrude2'''''''''''" cut sketch "Eclip_Groove" along normal blind 0.6 from surface at -89.6 bodies 26 in component "Hinge_Pin_D3_L"
sketch "Eclip_DIN6799_2.3_L" plane through (0, 0, 0) normal (1, 0, 0) x (0, 0, -1) in component "Eclip_DIN6799_2.3_L"
  circle A0 centre (102, 14.5) radius 3.5
  circle A1 centre (102, 14.5) radius 1.15
extrude "Extrude1''''''''''''''''''''''''''" add sketch "Eclip_DIN6799_2.3_L" along normal blind 0.6 from surface at -89.6 separate body makes body 27 in component "Eclip_DIN6799_2.3_L"
sketch "Wedgelet_Block_PETG_R" plane through (0, 0, 0) normal (1, 0, 0) x (0, 0, -1) in component "Wedgelet_Block_PETG_R"
  line L0 (100, 4) -> (100, 11)
  line L1 (100, 11) -> (104, 11)
  line L2 (104, 11) -> (104, 4)
  line L3 (104, 4) -> (100, 4)
extrude "Extrude1'''''''''''''''''''''''''''" add sketch "Wedgelet_Block_PETG_R" along normal blind 54 from surface at 34 separate body makes body 28 in component "Wedgelet_Block_PETG_R"
sketch "Knuckle (3)" plane through (0, 0, 0) normal (1, 0, 0) x (0, 0, -1) in component "Wedgelet_Block_PETG_R"
  line L0 (100, 11) -> (100, 16.5)
  line L1 (100, 16.5) -> (104, 16.5)
  line L2 (104, 16.5) -> (104, 11)
  line L3 (104, 11) -> (100, 11)
extrude "Extrude2''''''''''''" add sketch "Knuckle (3)" along normal blind 4 from surface at 34 bodies 28 in component "Wedgelet_Block_PETG_R"
sketch "Knuckle (1) (2)" plane through (0, 0, 0) normal (1, 0, 0) x (0, 0, -1) in component "Wedgelet_Block_PETG_R"
  line L0 (100, 11) -> (100, 16.5)
  line L1 (100, 16.5) -> (104, 16.5)
  line L2 (104, 16.5) -> (104, 11)
  line L3 (104, 11) -> (100, 11)
extrude "Extrude3'''''''''" add sketch "Knuckle (1) (2)" along normal blind 6 from surface at 60 bodies 28 in component "Wedgelet_Block_PETG_R"